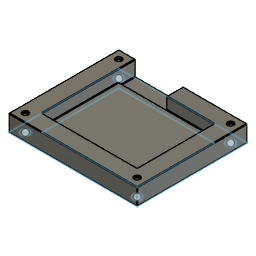
AudioVisualizerBase (Autodesk Fusion 360 design; units mm, degrees)
part number: 2025-12-05-15-46-46-018
Autodesk Fusion 360 part; units mm, degrees
sketch "Sketch1" plane through (0, 0, 0) normal (0, 1, 0) x (1, 0, 0)
  line L0 (5, 15) -> (61.65, 15)
  line L1 (61.65, 15) -> (61.65, -30.76)
  line L2 (61.65, -30.76) -> (5, -30.76)
  line L3 (5, -30.76) -> (5, 15)
  line L4 (-5, 25) -> (71.65, 25)
  line L5 (71.65, 25) -> (71.65, -40.76)
  line L6 (71.65, -40.76) -> (-5, -40.76)
  line L7 (-5, -40.76) -> (-5, 25)
  circle A0 centre (0, 20) radius 1.5
  circle A1 centre (66.65, 20) radius 1.5
  circle A2 centre (66.65, -35.76) radius 1.5
  circle A3 centre (0, -35.76) radius 1.5
  circle A4 centre (0, 20) radius 2.5
  circle A5 centre (66.65, 20) radius 2.5
  circle A6 centre (66.65, -35.76) radius 2.5
  circle A7 centre (0, -35.76) radius 2.5
  dimension "d1" = 56.65
  dimension "d2" = 45.76
  dimension "d3" = 65.76
  dimension "d4" = 10
  dimension "d5" = 76.65
  dimension "d6" = 10
  dimension "d7" = 3
  dimension "d8" = 3
  dimension "d9" = 3
  dimension "d10" = 3
  dimension "d11" = 5
  dimension "d12" = 5
  dimension "d13" = 5
  dimension "d14" = 5
  dimension "d15" = 5
  dimension "d16" = 5
  dimension "d17" = 5
  dimension "d18" = 5
  dimension "d19" = 5
  dimension "d20" = 5
  dimension "d21" = 5
  dimension "d22" = 5
  constraint horizontal L0
  constraint vertical L1
  constraint horizontal L2
  constraint vertical L3
  constraint horizontal L4
  constraint vertical L5
  constraint horizontal L6
  constraint vertical L7
  constraint concentric A0 A4
  constraint concentric A1 A5
  constraint concentric A2 A6
  constraint concentric A3 A7
  measures "d1" distance of L0.start L0.end
  measures "d2" distance of L0.start L2.end
  measures "d3" distance of L4.start L6.end
  measures "d4" distance of L0 L4
  measures "d5" distance of L4.start L4.end
  measures "d6" distance of L1 L5
  measures "d7" diameter of A0
  measures "d8" diameter of A1
  measures "d9" diameter of A2
  measures "d10" diameter of A3
  measures "d11" distance of L6 A3.centre
  measures "d12" distance of L7 A3.centre
  measures "d13" distance of L6 A2.centre
  measures "d14" distance of L5 A2.centre
  measures "d15" distance of L5 A1.centre
  measures "d16" distance of L4 A1.centre
  measures "d17" distance of L4 A0.centre
  measures "d18" distance of L7 A0.centre
  measures "d19" diameter of A4
  measures "d20" diameter of A5
  measures "d21" diameter of A6
  measures "d22" diameter of A7
extrude "Extrude1" add sketch "Sketch1" along normal blind 10 contours L4 L5 L6 L7 | A4 | A5 | A6 | A7
extrude "Extrude2" add sketch "Sketch1" along normal blind 9 contours A0 | A1 | A2 | A3
extrude "Extrude3" add sketch "Sketch1" along normal blind 3 contours L0 L1 L2 L3
sketch "Sketch2" plane through (0, 10, 0) normal (0, 1, 0) x (-1, 0, 0)
  circle A0 centre (-66.65, 35.76) radius 1.5
  circle A1 centre (0, 35.76) radius 1.5
  circle A2 centre (0, -20) radius 1.5
  circle A3 centre (-66.65, -20) radius 1.5
  line L0 (-61.65, 30.76) -> (-5, 30.76)
  line L1 (-5, 30.76) -> (-5, -15)
  line L2 (-5, -15) -> (-61.65, -15)
  line L3 (-61.65, -15) -> (-61.65, 30.76)
  line L4 (5, 40.76) -> (-71.65, 40.76)
  line L5 (-71.65, 40.76) -> (-71.65, -25)
  line L6 (-71.65, -25) -> (5, -25)
  line L7 (5, -25) -> (5, 40.76)
  line L8 (-5, -25) -> (-33.325, -25)
  line L9 (-33.325, -25) -> (-33.325, -15)
  line L10 (-33.325, -15) -> (-5, -15)
  line L11 (-5, -15) -> (-5, -25)
  constraint horizontal L8
  constraint vertical L9
  constraint horizontal L10
  constraint vertical L11
  constraint midpoint L2 L9.end
  constraint coincident L6 L8.start
extrude "Extrude4" cut sketch "Sketch2" against normal blind 9 contours L2 L6 L8 L9 L10 L11
fillet "Fillet1" radius 0.3 22 faces at (33.325, 3, 15.5067) (14.4417, 2.3333, -15) (20.55, 0, -3.08) (67.6974, 9.3333, -21.0738) (66.7613, 9, 36.2475) (33.325, 4.6667, -21.6667) (0.4727, 9, -19.6357) (67.5256, 9.3333, 34.5421) (-1.4981, 9.6667, -19.9252) (66.5387, 9, -20.4875) (5, 7.6667, -3.08) (46.1, 6.6667, 40.76) (-0.8158, 9, 35.5431) (58.875, 3.6667, -25) (42.7667, 5.3333, 30.76) (42.7667, 5.3333, -15) (-5, 6.6667, 18.84) (-1.3822, 9.6667, 36.3427) (61.65, 5.3333, 0.2533) (42.7667, 10, -18.3333) (23.8833, 1, -18.3333) (71.65, 6.6667, -3.08)
